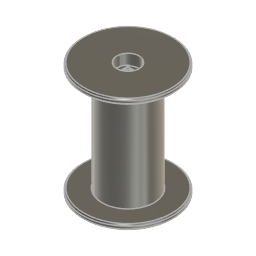
CapstanDrum_HGR (Autodesk Fusion 360 design; units mm, degrees)
Autodesk Fusion 360 part; units mm, degrees
sketch "Sketch1" plane through (0, 0, 0) normal (0, 0, 1) x (1, 0, 0)
  circle A0 centre (0, 0) radius 10.05
  line L0 (2.35, -4.25) -> (2.35, -9.45)
  line L1 (-2.35, -4.25) -> (2.35, -4.25)
  line L2 (-2.35, -4.25) -> (2.35, -9.45) construction
  line L3 (2.35, -9.45) -> (-2.35, -9.45)
  line L4 (2.35, -4.25) -> (-2.35, -9.45) construction
  line L5 (-2.35, -9.45) -> (-2.35, -4.25)
  circle A1 centre (0, 0) radius 7.15
  circle A2 centre (0, 0) radius 17.5
  line L6 (0, 0) -> (0, -12)
  point P0 (0, -6.85)
  dimension "d1" = 20.1
  dimension "d2" = 4.7
  dimension "d3" = 5.2
  dimension "d4" = 14.3
  dimension "d5" = 2.9
  dimension "d10" = 35
  constraint coincident A0.centre A1.centre
  constraint horizontal L1
  constraint perpendicular L0 L1
  constraint parallel L1 L3
  constraint parallel L0 L5
  constraint coincident P0 L2
  constraint coincident P0 L4
  constraint perpendicular L3 L6
  constraint coincident P0 L6
  measures "d1" diameter of A0
  measures "d2" distance of L3.end L0.end
  measures "d3" distance of L0.end L0.start
  measures "d4" diameter of A1
  measures "d5" distance of L1 A1
  measures "d10" diameter of A2
extrude "Extrude1" add sketch "Sketch1" along normal blind 42 contours A0 | L0 L1 A1 L6 | L0 L3 A1 L6 | L1 L5 A1 L6 | L3 L5 A1 L6 makes body 1
extrude "Extrude2" add sketch "Sketch1" along normal blind 2 contours A2 bodies 1
extrude "Extrude3" add sketch "Sketch1" along normal blind 2 from surface at 42 separate body contours A0 | L0 L1 A1 L6 | L0 L3 A1 L6 | L1 L5 A1 L6 | L3 L5 A1 L6 | A2 makes body 2
extrude "Extrude4" add sketch "Sketch1" against normal blind 20 from surface at 44 separate body contours L0 L1 L5 A1 | L0 L1 A1 L6 | L1 L5 A1 L6 makes body 3
combine "Combine1" operation add target body 2 tool bodies 3
move_face "OffsetFaces1" [suppressed]
sketch "Sketch2" plane through (0, 0, 44) normal (0, 0, 1) x (-1, 0, 0)
  circle A0 centre (0, 0) radius 17.5
  circle A1 centre (0, 0) radius 3
  constraint concentric A0 A1
extrude "Extrude5" cut sketch "Sketch1" against normal blind 18 from surface at 42 contours L0 L1 A1 L6 | L1 L5 A1 L6 bodies 1
hole "Hole1" at (0, 0, 44) direction (0, 0, -1) diameter 5.4 depth 65 tip angle 118 counterbore diameter 8.6 counterbore depth 4 bodies 2
extrude "Extrude6" cut sketch "Sketch1" along normal blind 7 contours L0 L1 A1 L6 | L1 L5 A1 L6 bodies 1
chamfer "Chamfer1" distance 2.5 angle 45 1 edges at (0, -4.25, 7) on bodies 1
move_face "OffsetFaces3" offset -0.1 1 faces at (7.1145, -0.7119, 36) on bodies 2
sketch "Sketch3" plane through (0, 0, 40) normal (0, 0, 1) x (-1, 0, 0)
  circle A0 centre (0, 0) radius 4.3
  circle A1 centre (0, 0) radius 2.7
  line L0 (-2.7, 2.7) -> (2.7, 2.7)
  line L1 (2.7, 2.7) -> (2.7, -2.7)
  line L2 (2.7, -2.7) -> (-2.7, -2.7)
  line L3 (-2.7, -2.7) -> (-2.7, 2.7)
  line L4 (-2.7, 2.7) -> (2.7, -2.7) construction
  line L5 (2.7, 2.7) -> (-2.7, -2.7) construction
  line L6 (2.7, -2.7) -> (2.7, -3.3466)
  line L7 (2.7, 2.7) -> (2.7, 3.3466)
  line L8 (-2.7, 2.7) -> (-2.7, 3.3466)
  line L9 (-2.7, -2.7) -> (-2.7, -3.3466)
  dimension "d33" = 5.4
  dimension "d34" = 5.4
  constraint horizontal L0
  constraint perpendicular L0 L1
  constraint parallel L0 L2
  constraint parallel L1 L3
  constraint coincident L4 A0.centre
  constraint coincident L5 A0.centre
  constraint coincident A0.centre A1.centre
  constraint coincident A0 L6.end
  constraint perpendicular L2 L6
  constraint coincident A0 L7.end
  constraint perpendicular L0 L7
  constraint coincident A0 L8.end
  constraint perpendicular L0 L8
  constraint coincident A0 L9.end
  constraint perpendicular L2 L9
  measures "d33" distance of L1.end L2.end
  measures "d34" distance of L0.end L1.end
extrude "Extrude8" cut sketch "Sketch3" against normal blind 0.2 contours A0 L0 L7 L8 | A0 L2 L6 L9 bodies 2
extrude "Extrude9" cut sketch "Sketch3" against normal blind 0.4 contours A1 L0 L1 | A1 L1 L2 | A1 L0 L3 | A1 L2 L3 bodies 2
chamfer "Chamfer2" distance 0.5 angle 45 7 edges at (-16.3157, -6.3283, 44) (-16.3157, 6.3283, 42) (-6.5729, 2.5494, 24) (-16.3157, -6.3283, 2) (-16.3157, -6.3283, 0) (-6.6661, 2.5856, 0) (-6.6661, 2.5856, 42) on bodies 1 2
